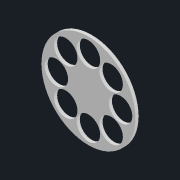
# Autodesk Inventor part: locating
Saved by Autodesk Inventor 2022.2 (Build 262287010, 287A)
## iProperties
Created: 2023-07-21
Part Number: locating
Material: Generic
Document SubType Name: Modeling
Designer: StijnC
Density: 1 g/cm^3
Appearance: Default
Author: StijnC
Autodesk Inventor part; units mm, degrees
ref_plane "YZ Plane" through (0, 0, 0) normal (1, 0, 0) x (0, 1, 0)
ref_plane "XZ Plane" through (0, 0, 0) normal (0, 1, 0) x (-1, 0, 0)
ref_plane "XY Plane" through (0, 0, 0) normal (0, 0, 1) x (1, 0, 0)
sketch "Sketch1" plane through (0, 0, 0) normal (0, 0, 1) x (1, 0, 0)
  circle A0 centre (-20.5, 0) radius 7.5
  circle A1 centre (-14.4957, -14.4957) radius 7.5
  circle A2 centre (0, -20.5) radius 7.5
  circle A3 centre (14.4957, -14.4957) radius 7.5
  circle A4 centre (20.5, 0) radius 7.5
  circle A5 centre (14.4957, 14.4957) radius 7.5
  circle A6 centre (0, 20.5) radius 7.5
  circle A7 centre (-14.4957, 14.4957) radius 7.5
  circle A8 centre (0, 0) radius 30
  dimension "d0" = 15
  dimension "d1" = 20.5
  dimension "d4" = 360
  dimension "d6" = 60
  constraints: 9 centre point, 1 coincident, 1 horizontal alignment, 17 other
  measures "d0" diameter of A0
  measures "d1" distance of point (0, 0) A0.centre
  measures "d6" diameter of A8
extrude "Extrusion1" add sketch "Sketch1" along normal blind 2
body "Solid1"
